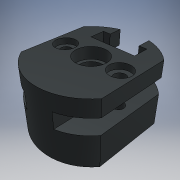
# Autodesk Inventor part: attachment
Saved by Autodesk Inventor 2018 (Build 220112000, 112)
## iProperties
Created: 2020-12-04
Part Number: attachment
Material: Všeobecné
Document SubType Name: Modeling
Designer: Jozko Mrkvicka
Density: 1 g/cm^3
Appearance: Výchozí
Author: Jozko Mrkvicka
Autodesk Inventor part; units mm, degrees
ref_plane "YZ Plane" through (0, 0, 0) normal (1, 0, 0) x (0, 1, 0)
ref_plane "XZ Plane" through (0, 0, 0) normal (0, 1, 0) x (-1, 0, 0)
sketch "Náčrt1" plane through (0, 0, 0) normal (0, 0, 1) x (1, 0, 0)
  line L0 (11, 8.6603) -> (11, -8.6603)
  line L1 (-11, -8.6603) -> (-11, 8.6603)
  arc A0 (-11, -8.6603) -> (11, -8.6603) centre (0, 0) ccw
  line L2 (-4, 13.4164) -> (-4, 10)
  line L3 (-4, 10) -> (-6, 10)
  line L4 (-6, 6) -> (6, 6)
  line L5 (6, 10) -> (4, 10)
  line L6 (4, 10) -> (4, 13.4164)
  line L7 (-6, 10) -> (-6, 6)
  line L8 (6, 10) -> (6, 6)
  arc A1 (11, 8.6603) -> (4, 13.4164) centre (0, 0) ccw
  arc A2 (-4, 13.4164) -> (-11, 8.6603) centre (0, 0) ccw
  dimension "d26" = 22
  dimension "attachmentRadius" = 14
  dimension "d28" = 14
  dimension "d29" = 14
  constraints: 18 end point, 6 point on circle, 4 perpendicular, 3 centre point, 2 horizontal alignment, 1 coincident, 1 parallel, 1 point on line, 1 vertical
  measures "d26" distance between parallel lines of L0 L1
  measures "attachmentRadius" radius of A0
  measures "d28" radius of A2
  measures "d29" radius of A1
extrude "Vysunutí1" add sketch "Náčrt1" along normal blind 20
ref_plane "Pracovní rovina1" through (0, 14, 0) normal (0, 1, 0) x (-1, 0, 0)
sketch "Náčrt2" plane through (0, 14, 0) normal (0, 1, 0) x (-1, 0, 0)
  line L0 (11, 0) -> (11, 20) projected
  line L1 (4, 0) -> (4, 20) projected
  line L2 (11, 16) -> (4, 16)
  line L3 (4, 16) -> (4, 12)
  line L4 (4, 12) -> (11, 12)
  line L5 (11, 12) -> (11, 16)
  line L6 (-4, 0) -> (-4, 20) projected
  line L7 (-11, 0) -> (-11, 20) projected
  line L8 (-4, 16) -> (-11, 16)
  line L9 (-11, 16) -> (-11, 12)
  line L10 (-11, 12) -> (-4, 12)
  line L11 (-4, 12) -> (-4, 16)
  point P0 (0, 0)
  constraints: 16 end point, 6 point on line, 4 parallel, 2 horizontal, 2 perpendicular
extrude "Vysunutí2" cut sketch "Náčrt2" against normal up to next
sketch "Náčrt6" plane through (0, 0, 20) normal (0, 0, 1) x (1, 0, 0)
  circle A0 centre (7.5, 0) radius 1.5
  circle A1 centre (-7.5, 0) radius 1.5
  line L0 (11, -8.6603) -> (11, 8.6603) projected
  line L1 (-11, 8.6603) -> (-11, -8.6603) projected
  arc A2 (11, 8.6603) -> (4, 13.4164) centre (0, 0) ccw projected
  dimension "d15" = 3.5
  dimension "attachmentHoleOffset" = 3.5
  dimension "d17" = 3
  dimension "attachmentHoleDia" = 3
  constraints: 2 centre point, 2 horizontal alignment
  measures "d15" distance from line of L0 A0.centre
  measures "attachmentHoleOffset" distance from line of A1.centre L1
  measures "d17" diameter of A0
  measures "attachmentHoleDia" diameter of A1
extrude "Vysunutí6" cut sketch "Náčrt6" against normal up to surface (20 mm away)
sketch "Náčrt8" plane through (0, 0, 0) normal (0, 0, -1) x (-1, 0, 0)
  circle A0 centre (-7.5, 0) radius 1.5 projected
  circle A1 centre (7.5, 0) radius 1.5 projected
  line L0 (-11, 8.6603) -> (-11, -8.6603) projected
  arc A2 (-11, -8.6603) -> (11, -8.6603) centre (0, 0) ccw projected
  line L1 (11, -8.6603) -> (11, 8.6603) projected
  arc A3 (11, 8.6603) -> (4, 13.4164) centre (0, 0) ccw projected
  line L2 (4, 13.4164) -> (4, 10) projected
  line L3 (4, 10) -> (6, 10) projected
  line L4 (6, 10) -> (6, 6) projected
  line L5 (6, 6) -> (-6, 6) projected
  line L6 (-6, 6) -> (-6, 10) projected
  line L7 (-6, 10) -> (-4, 10) projected
  line L8 (-4, 10) -> (-4, 13.4164) projected
  arc A4 (-4, 13.4164) -> (-11, 8.6603) centre (0, 0) ccw projected
extrude "Vysunutí8" cut sketch "Náčrt8" against normal blind 4
sketch "Náčrt9" plane through (0, 0, 20) normal (0, 0, 1) x (1, 0, 0)
  arc A0 (-4, 13.4164) -> (-11, 8.6603) centre (0, 0) ccw projected
  circle A1 centre (0, 0) radius 3
  constraints: 1 centre point, 1 coincident
extrude "Vysunutí9" cut sketch "Náčrt9" against normal up to next
sketch "Náčrt10" plane through (0, 0, 20) normal (0, 0, 1) x (1, 0, 0)
  circle A0 centre (0, 0) radius 3 projected
  arc A1 (-11, -8.6603) -> (11, -8.6603) centre (0, 0) ccw projected
  circle A2 centre (0, 0) radius 4
  dimension "d23" = 8
  constraints: 1 centre point, 1 coincident
  measures "d23" diameter of A2
extrude "Vysunutí10" cut sketch "Náčrt10" against normal blind 3
sketch "Náčrt11" plane through (0, 0, 20) normal (0, 0, 1) x (1, 0, 0)
  circle A0 centre (7.5, 0) radius 1.5 projected
  circle A1 centre (-7.5, 0) radius 1.5 projected
  circle A2 centre (-7.5, 0) radius 1.5 projected
  circle A3 centre (-7.5, 0) radius 2.75
  circle A4 centre (7.5, 0) radius 1.5 projected
  circle A5 centre (7.5, 0) radius 2.75
  dimension "d30" = 5.5
  dimension "d31" = 5.5
  constraints: 2 centre point, 2 coincident
  measures "d30" diameter of A3
  measures "d31" diameter of A5
extrude "Vysunutí11" cut sketch "Náčrt11" against normal blind 1.5
sketch "Náčrt12" plane through (0, 0, 4) normal (0, 0, -1) x (-1, 0, 0)
  line L0 (7.5, 3.1754) -> (10.25, 1.5877)
  line L1 (10.25, 1.5877) -> (10.25, -1.5877)
  line L2 (10.25, -1.5877) -> (7.5, -3.1754)
  line L3 (7.5, -3.1754) -> (4.75, -1.5877)
  line L4 (4.75, -1.5877) -> (4.75, 1.5877)
  line L5 (4.75, 1.5877) -> (7.5, 3.1754)
  line L6 (-11, -8.6603) -> (-11, 8.6603)
  circle A0 centre (-7.5, 0) radius 1.5 projected
  line L7 (-7.5, 3.1754) -> (-4.75, 1.5877)
  line L8 (-4.75, 1.5877) -> (-4.75, -1.5877)
  line L9 (-4.75, -1.5877) -> (-7.5, -3.1754)
  line L10 (-7.5, -3.1754) -> (-10.25, -1.5877)
  line L11 (-10.25, -1.5877) -> (-10.25, 1.5877)
  line L12 (-10.25, 1.5877) -> (-7.5, 3.1754)
  point P0 (7.5, 0)
  point P1 (7.5, 0)
  dimension "d38" = 5.5
  constraints: 26 end point, 2 coincident, 26 other
  measures "d38" distance between parallel lines of L8 L11
extrude "Vysunutí13" cut sketch "Náčrt12" against normal blind 2.4
equation "\"d28\" = attachmentRadius"
equation "\"d29\" = attachmentRadius"
equation "\"d15\" = attachmentHoleOffset"
equation "\"d17\" = attachmentHoleDia"
